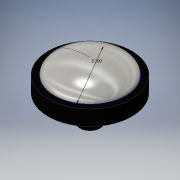
# Autodesk Inventor part: ButtonExtraLarge
Saved by Autodesk Inventor 2016 (Build 200138000, 138)
## iProperties
Created: 2017-01-21
Part Number: ButtonExtraLarge
Material: Generic
Document SubType Name: Modeling
Designer: Owner
Density: 1 g/cm^3
Appearance: Default
Author: Owner
Autodesk Inventor part; units mm, degrees
ref_plane "YZ Plane" through (0, 0, 0) normal (1, 0, 0) x (0, 1, 0)
ref_plane "XZ Plane" through (0, 0, 0) normal (0, 1, 0) x (-1, 0, 0)
ref_plane "XY Plane" through (0, 0, 0) normal (0, 0, 1) x (1, 0, 0)
sketch "Sketch1" plane through (0, 0, 0) normal (0, 1, 0) x (-1, 0, 0)
  line L0 (0, -68.453) -> (0, 68.453) projected
  line L1 (-68.453, 0) -> (68.453, 0) projected
  circle A0 centre (0, 0) radius 48.895
  dimension "d0" = 97.79
  constraints: 1 centre point, 1 coincident
  measures "d0" diameter of A0
extrude "Extrusion1" add sketch "Sketch1" along normal blind 17.78
sketch "Sketch2" plane through (0, 17.78, 0) normal (0, 1, 0) x (1, 0, 0)
  circle A0 centre (0, 0) radius 41.91
  dimension "d3" = 83.82
  constraints: 1 centre point, 1 coincident
  measures "d3" diameter of A0
sketch "Sketch3" plane through (0, 0, 0) normal (0, 0, 1) x (1, 0, 0)
  line L0 (41.91, 17.78) -> (-41.91, 17.78) projected
  ellipse E0 centre (0, 17.78) end of major axis (-41.91, 17.78) minor radius 17.78 (0, 35.56) -> (-41.91, 17.78) ccw
  line L1 (0, 35.56) -> (0, 17.78)
  line L2 (-41.91, 17.78) -> (0, 17.78)
  line L3 (0, 49.9292) -> (0, -8.3215) projected
  line L4 (-68.453, 0) -> (68.453, 0) projected
  point P0 (0, 0)
  dimension "d4" = 17.78
  constraints: 5 end point, 1 collinear, 1 horizontal, 1 midpoint, 1 point on line, 1 vertical, 5 other
revolve "Revolution2" add sketch "Sketch3" angle 360 about axis through (0, 0, 0) along (0, -1, 0)
sketch "Sketch4" plane through (0, 0, 0) normal (0, -1, 0) x (1, 0, 0)
  circle A0 centre (0, 0) radius 11.811
  dimension "d6" = 23.622
  constraints: 1 centre point, 1 coincident
  measures "d6" diameter of A0
extrude "Extrusion2" add sketch "Sketch4" along normal blind 30.48
body "Solid1"
